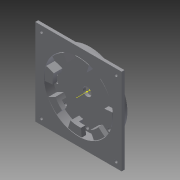
# Autodesk Inventor part: bayonet container 8
Saved by Autodesk Inventor 2015 (Build 190159000, 159)
## iProperties
Created: 2014-09-09
Part Number: bayonet container 8
Material: Generic
Document SubType Name: Modeling
Designer: ericd_000
Density: 1 g/cm^3
Appearance: Default
Author: ericd_000
Autodesk Inventor part; units mm, degrees
ref_plane "YZ Plane" through (0, 0, 0) normal (1, 0, 0) x (0, 1, 0)
ref_plane "XZ Plane" through (0, 0, 0) normal (0, 1, 0) x (-1, 0, 0)
ref_plane "XY Plane" through (0, 0, 0) normal (0, 0, 1) x (1, 0, 0)
sketch "Sketch1" plane through (0, 0, 0) normal (0, 1, 0) x (-1, 0, 0)
  line L0 (75, 75) -> (-75, 75)
  line L1 (-75, 75) -> (-75, -75)
  line L2 (-75, -75) -> (75, -75)
  line L3 (75, -75) -> (75, 75)
  circle A0 centre (0, 0) radius 35
  circle A1 centre (65, 65) radius 2.75
  circle A2 centre (-65, 65) radius 2.75
  circle A3 centre (-65, -65) radius 2.75
  circle A4 centre (65, -65) radius 2.75
  point P0 (75, 0)
  point P1 (0, -75)
  dimension "d0" = 150
  dimension "d1" = 150
  dimension "d2" = 70
  dimension "d3" = 5.5
  dimension "d4" = 10
  dimension "d5" = 10
  dimension "d8" = 360
  constraints: 8 end point, 5 centre point, 2 midpoint, 2 parallel, 1 coincident, 1 horizontal, 1 horizontal alignment, 1 perpendicular, 1 vertical alignment, 9 other
  measures "d0" distance of L2.end L0.start
  measures "d1" distance of L1.end L2.end
  measures "d2" diameter of A0
  measures "d3" diameter of A1
  measures "d4" distance from line of L3 A1.centre
  measures "d5" distance from line of L0 A1.centre
extrude "Extrusion1" add sketch "Sketch1" along normal blind 5
sketch "Sketch2" plane through (0, 0, 0) normal (0, -1, 0) x (1, 0, 0)
  circle A0 centre (0, 0) radius 65
  dimension "d12" = 130
  constraints: 1 centre point, 1 coincident
  measures "d12" diameter of A0
extrude "Extrusion2" cut sketch "Sketch2" against normal blind 10
sketch "Sketch3" plane through (0, 0, 0) normal (0, -1, 0) x (1, 0, 0)
  circle A0 centre (0, 0) radius 65
  circle A1 centre (0, 0) radius 60
  dimension "d15" = 130
  dimension "d16" = 120
  constraints: 2 centre point, 2 coincident
  measures "d15" diameter of A0
  measures "d16" diameter of A1
extrude "Extrusion3" add sketch "Sketch3" against normal blind 20
sketch "Sketch4" plane through (0, 20, 0) normal (0, 1, 0) x (1, 0, 0)
  circle A0 centre (0, 0) radius 60
  point P0 (0, 0)
  dimension "d42" = 120
  constraints: 1 centre point, 1 coincident
  measures "d42" diameter of A0
extrude "Extrusion4" add sketch "Sketch4" against normal blind 5
sketch "Sketch5" plane through (0, 15, 0) normal (0, -1, 0) x (1, 0, 0)
  circle A0 centre (0, 54) radius 3
  point P0 (0, 0)
  dimension "d21" = 6
  dimension "d22" = 54
  constraints: 1 centre point
  measures "d21" diameter of A0
  measures "d22" distance of A0.centre point (0, 0)
extrude "Extrusion5" cut sketch "Sketch5" against normal through all
pattern_circular "Circular Pattern1" count 8 over 360 about axis through (0, 0, 0) along (0, 1, 0) of "Extrusion5"
sketch "Sketch6" plane through (0, 15, 0) normal (0, -1, 0) x (1, 0, 0)
  circle A0 centre (0, 0) radius 7.5
  point P0 (0, 0)
  dimension "d28" = 15
  constraints: 1 centre point, 1 coincident
  measures "d28" diameter of A0
extrude "Extrusion6" cut sketch "Sketch6" against normal blind 10
sketch "Sketch7" plane through (0, 15, 0) normal (0, -1, 0) x (1, 0, 0)
  circle A0 centre (0, 0) radius 45
  circle A1 centre (0, 0) radius 60 projected
  line L0 (0, 0) -> (-26.7546, 36.1827) construction
  circle A2 centre (-38.1838, 38.1838) radius 3 projected
  line L1 (0, 0) -> (-20.4478, 40.086) construction
  circle A3 centre (0, 0) radius 59
  line L2 (-20.4478, 40.086) -> (-26.8093, 52.5572)
  line L3 (-26.7546, 36.1827) -> (-35.0783, 47.4396)
  point P0 (-38.3158, 46.1725)
  point P1 (-27.2637, 53.448)
  dimension "d31" = 15
  dimension "d43" = 120
  dimension "d44" = 118
  dimension "d45" = 14
  dimension "d66" = 8
  dimension "d67" = 170.546
  constraints: 8 end point, 6 point on circle, 2 centre point, 2 coincident, 2 collinear, 1 point on line
  measures "d31" radial gap between concentric circles of A1 A0
  measures "d43" diameter of A1
  measures "d44" diameter of A3
  measures "d45" radial gap between concentric circles of A3 A0
  measures "d66" distance from line of L3 A2.centre
  measures "d67" angle of L2 L3
extrude "Extrusion7" add sketch "Sketch7" along normal blind 15 contours A0 L3 A3 L2 picked at (-30.7402, 44.7782)
sketch "Sketch9" plane through (0, 0, 0) normal (0, -1, 0) x (1, 0, 0)
  circle A0 centre (0, 0) radius 29.9834
  circle A1 centre (0, 0) radius 39.9778
  line L0 (0, 0) -> (-26.8767, 13.2908) construction
  line L1 (-35.8356, 17.721) -> (-26.8767, 13.2908)
  point P0 (0, 0)
  constraints: 4 end point, 2 coincident, 1 collinear, 1 point on line, 6 other
sketch "Sketch10" plane through (-26.7546, 0, 36.1827) normal (-0.8040605, 0, -0.5945474) x (-0.5945474, 0, 0.8040605)
  line L0 (0, 0) -> (14, 0)
  line L1 (14, 0) -> (14, 7.5)
  line L2 (14, 15) -> (14, 0) projected
  line L3 (0, 15) -> (0, 0) projected
  line L4 (0, 7.5) -> (14, 7.5)
  line L5 (0, 15) -> (14, 15)
  line L6 (-45, -4) -> (-45, 24) projected
  point P0 (-45, 0)
  dimension "d46" = 7.5
  constraints: 8 end point, 2 horizontal, 2 midpoint, 1 parallel
  measures "d46" distance between parallel lines of L0 L4
revolve "Revolution2" add sketch "Sketch10" angle 14 about axis through (0, 0, 0) along (0, -1, 0) contours L3 L4 L1 L0
sketch "Sketch11" plane through (0, 0, 0) normal (0, -1, 0) x (1, 0, 0)
  line L0 (-34.7133, 28.6354) -> (-45.513, 37.5442) projected
  arc A0 (-20.4478, 40.086) -> (-20.4478, 40.086) centre (0, 0) ccw projected
  line L1 (-40.1131, 33.0898) -> (-34.7133, 28.6354)
  line L2 (-30.497, 33.0898) -> (-40.1131, 33.0898)
  line L3 (-30.497, 33.0898) -> (-34.7133, 28.6354)
  point P0 (0, 0)
  constraints: 6 end point, 1 collinear, 1 horizontal, 1 midpoint, 2 other
pattern_circular "Circular Pattern2" count 8 over 360 about axis through (0, 0, 0) along (0, 1, 0) of "Extrusion7", "Revolution2"
sketch "Sketch12" plane through (0, 0, 0) normal (0, -1, 0) x (0.7798497, 0, 0.6259668)
  line L0 (-50.9146, -10.5691) -> (-44.0607, -9.1463)
  line L1 (-44.0607, -9.1463) -> (-57.7685, -11.9919) projected
  arc A0 (-44.8909, -3.1319) -> (-44.0607, -9.1463) centre (0, 0) ccw
  arc A1 (-44.0607, 9.1463) -> (-44.0607, 9.1463) centre (0, 0) ccw projected
  line L2 (-50.9146, -10.5691) -> (-44.8909, -3.1319)
  line L3 (-50.9146, -10.5691) -> (-44.8909, -3.1319) projected
  point P0 (0, 0)
  constraints: 4 end point, 2 collinear, 2 point on circle, 1 centre point, 2 other
extrude "Extrusion9" add sketch "Sketch12" against normal up to surface (7.5 mm away) contours L2 A0 L0
sketch "Sketch13" plane through (0, 20, 0) normal (0, 1, 0) x (1, 0, 0)
  circle A0 centre (0, 0) radius 65
  circle A1 centre (0, 0) radius 61
  dimension "d52" = 4
  dimension "d53" = 130
  constraints: 2 centre point, 2 coincident
  measures "d52" radial gap between concentric circles of A0 A1
  measures "d53" diameter of A0
extrude "Extrusion10" add sketch "Sketch13" along normal blind 13
sketch "Sketch17" plane through (0, 0, 0) normal (0, 0, 1) x (1, 0, 0)
  line L0 (61, 20) -> (-61, 20) projected
  line L1 (61.0173, 20) -> (-61, 20)
  line L2 (-61, 20) -> (-61, 51.3289)
  line L3 (-61, 51.3289) -> (61.0173, 51.3289)
  line L4 (61.0173, 51.3289) -> (61.0173, 20)
  point P0 (0, 0)
  constraints: 8 end point, 2 parallel, 1 horizontal, 1 perpendicular, 1 point on line
extrude "Extrusion13" cut sketch "Sketch17" along normal through all both and the other way through all
sketch "Sketch14" plane through (0, 33, 0) normal (0, 1, 0) x (1, 0, 0)
  circle A0 centre (0, 0) radius 65
  constraints: 1 centre point, 1 coincident
extrude "Extrusion11" add sketch "Sketch14" along normal blind 5
sketch "Sketch18" plane through (0, 20, 0) normal (0, 1, 0) x (1, 0, 0)
  point P0 (0, 0)
sketch "Sketch19" plane through (0, 33, 0) normal (0, -1, 0) x (1, 0, 0)
  circle A0 centre (0, 0) radius 6
  dimension "d63" = 12
  constraints: 1 centre point, 1 coincident
  measures "d63" diameter of A0
extrude "Extrusion14" add sketch "Sketch19" along normal blind 2
sketch "Sketch20" plane through (0, 15, 0) normal (0, -1, 0) x (1, 0, 0)
  circle A0 centre (-38.1838, 38.1838) radius 3
  circle A1 centre (-38.1838, 38.1838) radius 3 projected
  point P0 (0, 0)
  dimension "d68" = 6
  constraints: 1 centre point, 1 concentric
  measures "d68" diameter of A0
extrude "Extrusion15" cut sketch "Sketch20" against normal through all
pattern_circular "Circular Pattern3" count 8 over 360 about axis through (0, 0, 0) along (0, 1, 0) of "Extrusion15"
extrude "Extrusion16" cut sketch "Sketch11" against normal blind 10 contours L0 L2 A0 | A0 L3 picked at (-32.8621, 30.6363)
sketch "Sketch21" plane through (0, 0, 0) normal (0, 0, 1) x (1, 0, 0)
  line L0 (79.7641, 55.8787) -> (-85.0233, 55.8787)
  line L1 (-85.0233, 55.8787) -> (-85.0233, 20)
  line L2 (-85.0233, 20) -> (79.7641, 20)
  line L3 (79.7641, 20) -> (79.7641, 55.8787)
  point P0 (0, 0)
  constraints: 8 end point, 2 parallel, 1 horizontal, 1 perpendicular
extrude "Extrusion17" cut sketch "Sketch21" along normal through all both and the other way through all
sketch "Sketch23" plane through (0, 15, 0) normal (0, -1, 0) x (1, 0, 0)
  circle A0 centre (-52.6667, -11.9257) radius 1.5
  circle A1 centre (11.9257, -52.6667) radius 1.5
  circle A2 centre (52.6667, 11.9257) radius 1.5
  circle A3 centre (-11.9257, 52.6667) radius 1.5
  circle A4 centre (54, 0) radius 3 projected
  point P0 (0, 0)
  dimension "d79" = 3
  dimension "d82" = 360
  dimension "d93" = 12
  dimension "d94" = 54
  constraints: 4 centre point, 9 other
  measures "d79" diameter of A0
  measures "d93" distance of A4.centre A2.centre
  measures "d94" distance of point (0, 0) A0.centre
extrude "Extrusion18" cut sketch "Sketch23" against normal through all contours A0 | A1 | A2 | A3
sketch "Sketch24" plane through (0, 15, 0) normal (0, -1, 0) x (1, 0, 0)
  circle A0 centre (52.6667, 11.9257) radius 2.5
  circle A1 centre (52.6667, 11.9257) radius 1.5 projected
  circle A2 centre (-11.9257, 52.6667) radius 2.5
  circle A3 centre (-52.6667, -11.9257) radius 2.5
  circle A4 centre (11.9257, -52.6667) radius 2.5
  point P0 (0, 0)
  dimension "d86" = 5
  dimension "d89" = 360
  constraints: 4 centre point, 1 concentric, 9 other
  measures "d86" diameter of A0
extrude "Extrusion19" cut sketch "Sketch24" against normal blind 2
sketch "Sketch25" plane through (0, 15, 0) normal (0, -1, 0) x (1, 0, 0)
  point P0 (0, 0)
body "Solid1"
